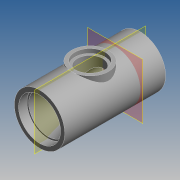
# Autodesk Inventor part: P007_CanonSupportRervoir
Saved by Autodesk Inventor 2020 (Build 240168000, 168)
## iProperties
Created: 2021-10-15
Part Number: P007_CanonSupportRervoir
Material: Générique
Document SubType Name: Modeling
Designer: gabri
Density: 1 g/cm^3
Appearance: Par défaut
Author: gabri
Autodesk Inventor part; units mm, degrees
sketch "Esquisse2" plane through (0, 0, 0) normal (0, 0, 1) x (1, 0, 0)
  line L0 (0, 16.6667) -> (0, -18.8492)
  line L1 (0, 54) -> (0, -114) construction
  line L2 (30, 30) -> (25, 30)
  line L3 (25, 30) -> (25, 20)
  line L4 (25, 20) -> (23, 20)
  line L5 (23, 20) -> (15, 0)
  line L6 (15, 0) -> (15, -60)
  line L7 (15, -60) -> (23, -80)
  line L8 (23, -80) -> (25, -80)
  line L9 (25, -80) -> (25, -90)
  line L10 (25, -90) -> (30, -90)
  line L11 (30, -90) -> (30, 30)
  line L12 (-6, 0) -> (36, 0) construction
  dimension "d4" = 30
  dimension "d5" = 50
  dimension "d6" = 60
  dimension "d8" = 10
  dimension "d9" = 100
  dimension "d10" = 30
  dimension "d11" = 10
  dimension "d12" = 2
  dimension "d13" = 2
  dimension "d14" = 20
  dimension "d15" = 20
  dimension "d17" = 21.801
  constraints: 22 end point, 4 perpendicular, 3 point on line, 2 parallel, 1 horizontal, 1 vertical
  measures "d4" diameter of L6 L0
  measures "d5" diameter of L3 L0
  measures "d6" diameter of L11 L0
  measures "d8" distance of L2.end L3.end
  measures "d9" distance between parallel lines of L8 L4
  measures "d10" distance between parallel lines of L12 L2
  measures "d11" distance of L8.end L9.end
  measures "d12" distance of L3.end L4.end
  measures "d13" distance of L7.end L8.end
  measures "d14" vertical distance of L4.end L5.end
  measures "d15" vertical distance of L6.end L7.end
  measures "d17" angle of L3 L5
revolve "Révolution1" add sketch "Esquisse2" angle 360 about axis through (0, 16.6667, 0) along (0, -1, 0)
ref_plane "Plan de construction1" through (0, 0, 30) normal (0, 0, 1) x (1, 0, 0)
sketch "Esquisse3" plane through (0, 0, 30) normal (0, 0, 1) x (1, 0, 0)
  line L0 (-15, -60) -> (15, -60) construction
  line L1 (-15, 0) -> (-23, 20) construction
  line L2 (15, 0) -> (23, 20) construction
  line L3 (-32.34, 0) -> (32.34, 0) construction
  line L4 (-23, -80) -> (-15, -60) construction
  line L5 (23, -80) -> (15, -60) construction
  circle A0 centre (0, -30) radius 15
  line L6 (0, 40) -> (0, -100) construction
  line L7 (-15, -60) -> (-15, 0) construction
  line L8 (15, -60) -> (15, 0) construction
  point P0 (0, 0)
  dimension "d19" = 60
  dimension "d20" = 30
  dimension "d21" = 30
  constraints: 1 centre point, 1 midpoint
  measures "d19" distance between parallel lines of L3 L0
  measures "d20" diameter of A0
  measures "d21" distance from line of L3 A0.centre
extrude "Extrusion1" cut sketch "Esquisse3" against normal blind 30
sketch "Esquisse4" plane through (0, 0, 30) normal (0, 0, 1) x (1, 0, 0)
  arc A0 (15, -30) -> (-15, -30) centre (0, -30) ccw construction
  arc A1 (-15, -30) -> (15, -30) centre (0, -30) ccw construction
  line L0 (-15, -60) -> (15, -60) construction
  line L1 (-15, 0) -> (15, 0) construction
  circle A2 centre (0, -30) radius 22
  circle A3 centre (0, -30) radius 15
  point P0 (0, 0)
  point P1 (0, -15)
  point P2 (0, -45)
  dimension "d24" = 44
  constraints: 3 vertical alignment, 2 coincident, 1 centre point, 2 other
  measures "d24" diameter of A2
extrude "Extrusion2" add sketch "Esquisse4" against normal blind 10
sketch "Esquisse6" plane through (0, 0, 30) normal (0, 0, 1) x (1, 0, 0)
  circle A0 centre (0, -30) radius 15 construction
  arc A1 (0, -8) -> (0, -52) centre (0, -30) ccw construction
  arc A2 (0, -52) -> (0, -8) centre (0, -30) ccw construction
  circle A3 centre (0, -30) radius 15
  circle A4 centre (0, -30) radius 18
  point P0 (0, 0)
  dimension "d27" = 36
  constraints: 2 centre point, 2 coincident, 1 concentric
  measures "d27" diameter of A4
extrude "Extrusion3" cut sketch "Esquisse6" against normal blind 5
